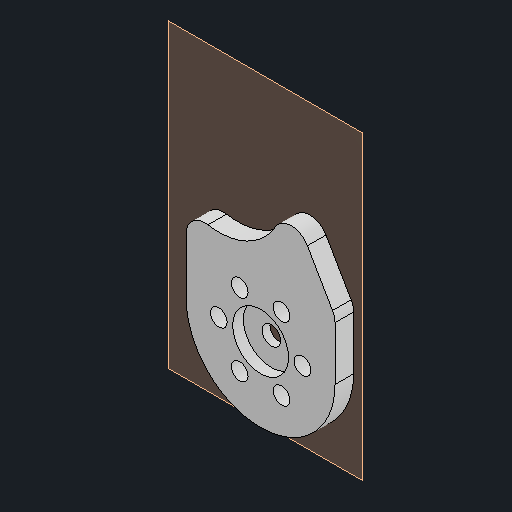
# Autodesk Inventor part: Motor_Mount
Saved by Autodesk Inventor 2024.2 (Build 282272000, 272)
## iProperties
Created: 2024-01-10
Part Number: Motor_Mount
Material: 一般
Document SubType Name: Modeling
Designer: Hanaoka
Density: 1 g/cm^3
Appearance: 既定
Author: Hanaoka
Autodesk Inventor part; units mm, degrees
ref_plane "YZ Plane" through (0, 0, 0) normal (1, 0, 0) x (0, 1, 0)
ref_plane "XZ Plane" through (0, 0, 0) normal (0, 1, 0) x (-1, 0, 0)
ref_plane "XY Plane" through (0, 0, 0) normal (0, 0, 1) x (1, 0, 0)
ref_plane "作業平面1" through (0, 0, 0) normal (0, 0, 1) x (1, 0, 0)
sketch "スケッチ1" plane through (0, 0, 0) normal (0, 0, 1) x (1, 0, 0)
  arc A0 (-6.5014, -6.7164) -> (9.4986, -6.7164) centre (1.4986, -6.7164) ccw projected
  line L0 (9.4986, -6.7164) -> (9.4986, -0.9651) projected
  arc A1 (9.4986, -0.9651) -> (9.2306, 0.0349) centre (7.4986, -0.9651) ccw projected
  line L1 (9.2306, 0.0349) -> (2.6306, 11.4664) projected
  arc A2 (2.6306, 11.4664) -> (-8.6277, 4.9664) centre (-2.9986, 8.2164) ccw projected
  line L2 (-8.6277, 4.9664) -> (-6.9034, 1.9797) projected
  arc A3 (-6.5014, 0.4797) -> (-6.9034, 1.9797) centre (-9.5014, 0.4797) ccw projected
  line L3 (-6.5014, 0.4797) -> (-6.5014, -6.7164) projected
  circle A4 centre (-2.9986, 8.2164) radius 3 projected
  circle A5 centre (1.4986, -6.7164) radius 1 projected
  circle A6 centre (5.9986, -6.7164) radius 0.9
  line L4 (5.9986, -6.7164) -> (1.4986, -6.7164) construction
  circle A7 centre (3.7486, -2.8193) radius 0.9
  circle A8 centre (-0.7514, -2.8193) radius 0.9
  circle A9 centre (-3.0014, -6.7164) radius 0.9
  circle A10 centre (-0.7514, -10.6135) radius 0.9
  circle A11 centre (3.7486, -10.6135) radius 0.9
  circle A12 centre (1.4986, -6.7164) radius 3
  arc A13 (-6.5014, 2.1559) -> (3.9296, 9.2164) centre (-2.9986, 8.2164) ccw
  circle A14 centre (1.4986, -6.7164) radius 1
  line L5 (-6.5014, 2.1559) -> (-6.5014, 0.4797)
  point P0 (0, 0)
  dimension "d0" = 4.5
  dimension "d1" = 1.8
  dimension "d4" = 360
  dimension "d6" = 6
  dimension "d7" = 7
  dimension "d10" = 2
  constraints: 9 centre point, 4 coincident, 4 end point, 2 point on circle, 2 point on line, 1 horizontal, 13 other
  measures "d0" distance of L4.start L4.end
  measures "d1" diameter of A6
  measures "d6" diameter of A12
  measures "d7" radius of A13
  measures "d10" diameter of A14
extrude "押し出し1" add sketch "スケッチ1" along normal blind 2 contours L3 L5 A13 L1 A1 L0 A0 | A12
sketch "スケッチ2" plane through (0, 0, 2) normal (0, 0, 1) x (1, 0, 0)
  line L0 (9.2306, 0.0349) -> (3.9296, 9.2164) projected
  line L1 (-6.5014, 2.1559) -> (-6.5014, -6.7164) projected
  arc A0 (-6.5014, -6.7164) -> (9.4986, -6.7164) centre (1.4986, -6.7164) ccw projected
  line L2 (9.4986, -6.7164) -> (9.4986, -0.9651) projected
  arc A1 (9.4986, -0.9651) -> (9.2306, 0.0349) centre (7.4986, -0.9651) ccw projected
  circle A2 centre (3.7486, -10.6135) radius 0.9 projected
  circle A3 centre (-0.7514, -10.6135) radius 0.9 projected
  circle A4 centre (-3.0014, -6.7164) radius 0.9 projected
  circle A5 centre (-0.7514, -2.8193) radius 0.9 projected
  circle A6 centre (3.7486, -2.8193) radius 0.9 projected
  circle A7 centre (5.9986, -6.7164) radius 0.9 projected
  circle A8 centre (1.4986, -6.7164) radius 1 projected
  circle A9 centre (1.4986, -6.7164) radius 3
  arc A10 (-6.5014, 2.1559) -> (3.9296, 9.2164) centre (-2.9986, 8.2164) ccw projected
  point P0 (0, 0)
  dimension "d11" = 6
  constraints: 1 centre point, 1 coincident
  measures "d11" diameter of A9
extrude "押し出し2" cut sketch "スケッチ2" against normal blind 1.15 contours A9
fillet "フィレット1" radius 2 2 edges at (3.9296, 9.2164, 1) (-6.5014, 2.1559, 1)
